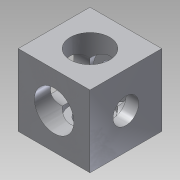
# Autodesk Inventor part: Corner Connector - Three Way Cube
Saved by Autodesk Inventor 2013 SP2 (Build 170200200, 200)
## iProperties
Created: 2013-06-26
Part Number: Corner Connector - Three Way Cube
Material: Aluminum 6061
Document SubType Name: Modeling
Designer: Jon Hollander
Density: 2.71 g/cm^3
Mass: 12.8935 g
Surface Area: 30.7917 cm^2
Volume: 4.75776 cm^3
Author: Jon Hollander
Autodesk Inventor part; units mm, degrees
ref_plane "YZ Plane" through (0, 0, 0) normal (1, 0, 0) x (0, 1, 0)
ref_plane "XZ Plane" through (0, 0, 0) normal (0, 1, 0) x (-1, 0, 0)
ref_plane "XY Plane" through (0, 0, 0) normal (0, 0, 1) x (1, 0, 0)
sketch "Sketch1" plane through (0, 0, 0) normal (0, 0, 1) x (1, 0, 0)
  line L0 (0, 0) -> (20, 0)
  line L1 (20, 0) -> (20, 20)
  line L2 (20, 20) -> (0, 20)
  line L3 (0, 20) -> (0, 0)
  dimension "d0" = 20
  dimension "d1" = 20
  constraints: 8 end point, 2 parallel, 1 horizontal, 1 perpendicular
  measures "d0" distance of L2.end L1.end
  measures "d1" distance of L1.end L0.end
extrude "Extrusion1" add sketch "Sketch1" along normal blind 20
sketch "Sketch2" plane through (0, 0, 20) normal (0, 0, 1) x (1, 0, 0)
  circle A0 centre (10, 10) radius 3.57
  circle A1 centre (10, 10) radius 5.5
  dimension "d4" = 7.14
  dimension "d5" = 11
  constraints: 2 centre point, 1 coincident
  measures "d4" diameter of A0
  measures "d5" diameter of A1
extrude "Extrusion2" cut sketch "Sketch2" against normal through all contours A0
extrude "Extrusion3" cut sketch "Sketch2" against normal blind 16.5
sketch "Sketch3" plane through (0, 20, 0) normal (0, 1, 0) x (1, 0, 0)
  line L0 (20, 0) -> (0, 0) projected
  line L1 (0, 0) -> (0, -20) projected
  line L2 (20, -20) -> (0, -20) projected
  line L3 (20, 0) -> (20, -20) projected
  point P0 (10, -10)
sketch "Sketch4" plane through (20, 0, 0) normal (1, 0, 0) x (0, 0, -1)
  line L0 (0, 0) -> (0, 20) projected
  line L1 (0, 20) -> (-20, 20) projected
  line L2 (-20, 0) -> (-20, 20) projected
  line L3 (0, 0) -> (-20, 0) projected
  point P0 (-10, 10)
pattern_circular "Circular Pattern1" count 2 over 90 about axis through (20, 10, 10) along (1, 0, 0) of "Extrusion3", "Extrusion2"
pattern_circular "Circular Pattern2" count 2 over 90 about axis through (10, 20, 10) along (0, -1, 0) of "Extrusion2", "Extrusion3"
body "Solid1"
